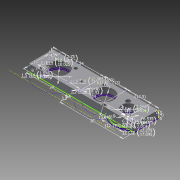
# Autodesk Inventor part: mount
Saved by Autodesk Inventor 2014 (Build 180170000, 170)
## iProperties
Created: 2013-09-13
Part Number: mount
Material: Generic
Document SubType Name: Modeling
Designer: Brandon
Density: 1 g/cm^3
Appearance: Default
Author: Brandon
Autodesk Inventor part; units mm, degrees
ref_plane "YZ Plane" through (0, 0, 0) normal (1, 0, 0) x (0, 1, 0)
ref_plane "XZ Plane" through (0, 0, 0) normal (0, 1, 0) x (-1, 0, 0)
ref_plane "XY Plane" through (0, 0, 0) normal (0, 0, 1) x (1, 0, 0)
sketch "Sketch1" plane through (0, 0, 0) normal (0, 0, 1) x (1, 0, 0)
  circle A0 centre (0, 0) radius 0.88
  circle A1 centre (-13, 0) radius 6.031
  line L0 (0, 7.8745) -> (0, -6.1255)
  line L1 (-24, -6.1255) -> (0, -6.1255)
  line L2 (-24, 7.8745) -> (-24, -6.1255)
  circle A2 centre (-13, 0) radius 5.1925
  line L3 (-13, 0) -> (-9.1435, 0) construction
  line L4 (-13, 0) -> (-13, 0) construction
  circle A3 centre (-8.099, 4.901) radius 0.8125
  circle A4 centre (-17.901, -4.901) radius 0.8125
  circle A5 centre (13, 0) radius 6.031
  circle A6 centre (13, 0) radius 5.1925
  line L5 (13, 0) -> (9.1435, 0) construction
  line L6 (13, 0) -> (13, 0) construction
  circle A7 centre (8.099, 4.901) radius 0.8125
  circle A8 centre (17.901, -4.901) radius 0.8125
  line L7 (13, 0) -> (-13, 0)
  circle A9 centre (26.5, 0) radius 4.5 construction
  circle A10 centre (26.5, 0) radius 8.6375
  line L8 (26.5, 0) -> (30.5894, 0) construction
  circle A11 centre (22.8938, 3.6062) radius 1.132
  circle A12 centre (30.1062, -3.6062) radius 1.132
  line L9 (0, -6.1255) -> (-0.0048, -7.7255) construction
  line L10 (-0.0048, -7.7255) -> (-19.5613, -7.6674) construction
  line L11 (-0.0048, -7.7255) -> (19.5518, -7.7836) construction
  circle A13 centre (13, 0) radius 9 construction
  circle A14 centre (26.5, 0) radius 2.5 construction
  circle A15 centre (26.5, 0) radius 3.2675
  line L12 (13, 0) -> (26.5, 0)
  line L13 (30.1062, -3.6062) -> (22.8938, 3.6062) construction
  line L14 (33.2882, -0.4243) -> (26.0757, 6.7882)
  line L15 (19.7118, 0.4243) -> (26.9243, -6.7882)
  arc A16 (26.9243, -6.7882) -> (33.2882, -0.4243) centre (30.1062, -3.6062) ccw
  arc A17 (26.0757, 6.7882) -> (19.7118, 0.4243) centre (22.8938, 3.6062) ccw
  circle A18 centre (26.5, 0) radius 7.7
  circle A19 centre (26.5, 0) radius 3.5
  line L16 (-24, 7.8745) -> (0, 7.8745)
  line L17 (36, 7.8745) -> (36, -6.1255)
  line L18 (20.4103, -6.1255) -> (32.5897, -6.1255) construction
  line L19 (-0.0048, -7.7255) -> (0.0011, -10.9255) construction
  line L20 (0.0011, -10.9255) -> (30.0189, -10.8709) construction
  line L21 (0.0011, -10.9255) -> (-29.9989, -10.9801) construction
  line L22 (0.0011, -10.9255) -> (30.001, -10.9255) construction
  circle A20 centre (0, 0) radius 4 construction
  line L23 (-13, 0) -> (-8.7354, 4.2646) construction
  line L24 (-13, 0) -> (-17.2646, -4.2646) construction
  line L25 (-8.7354, 4.2646) -> (-8.099, 4.901) construction
  line L26 (-17.2646, -4.2646) -> (-17.901, -4.901) construction
  line L27 (-17.2646, -4.2646) -> (-16.3646, -4.2646) construction
  circle A21 centre (13, 0) radius 12 construction
  circle A22 centre (-13, 0) radius 12 construction
  line L28 (1, 0) -> (-1, 0) construction
  line L29 (-19.031, 0) -> (-24, 0) construction
  line L30 (18.7135, -4.901) -> (18.7135, 10.099) construction
  line L31 (21.7618, 3.6062) -> (21.7618, -11.3938) construction
  line L32 (18.7135, -4.2879) -> (21.7618, -4.2879) construction
  line L33 (0, 7.8745) -> (36, 7.8745)
  line L34 (0, -6.1255) -> (36, -6.1255)
  dimension "d31" = 2
  dimension "d105" = 24
  dimension "d106" = 24
  dimension "d0" = 1.5
  dimension "d3" = 11.6
  dimension "d8" = 10
  dimension "d14" = 1.5
  dimension "d26" = 17
  dimension "d32" = 2
  dimension "d38" = 5
  dimension "d40" = 6.15
  dimension "d42" = 13
  dimension "d52" = 13.5
  dimension "d53" = 9
  dimension "d54" = 7
  dimension "d60" = 12.1794
  dimension "d81" = 1.6
  dimension "d86" = 3.2
  dimension "d87" = 45
  dimension "d88" = 10.2
  dimension "d89" = 8
  dimension "d91" = 0.9
  dimension "d92" = 135
  dimension "d98" = 14
  dimension "d103" = 18
  dimension "d104" = 9
  dimension "d107" = 2
  dimension "d108" = 4.969
  dimension "d114" = 3.0483
  dimension "d117" = 24
  dimension "d118" = 24
  dimension "d119" = 36
  constraints: 72 end point, 19 centre point, 15 coincident, 10 horizontal, 9 point on circle, 9 point on line, 7 collinear, 7 perpendicular, 6 symmetric about line, 6 tangent, 4 horizontal alignment, 3 equal length, 2 midpoint, 2 vertical, 1 equal radius, 1 parallel, 12 other
  measures "d38" diameter of A14
  measures "d42" distance of point (0, 0) A5.centre
  measures "d52" distance of L12.start L8.start
  measures "d53" diameter of A17
  measures "d54" diameter of A19
  measures "d60" distance of L18.start L18.end
  measures "d81" distance of L9.end L0.end
  measures "d86" distance of L9.end L19.end
  measures "d87" angle of L8 L13
  measures "d88" distance of L13.start L13.end
  measures "d89" diameter of A20
  measures "d91" distance of L24.end L26.end
  measures "d92" angle of L26 L27
  measures "d98" distance of L2.start L1.start
  measures "d103" diameter of A13
  measures "d104" diameter of A9
  measures "d107" distance of L28.start L28.end
  measures "d108" distance of L29.start L29.end
  measures "d114" distance of L32.start L32.end
  measures "d117" distance of L2.start L0.start
  measures "d118" distance of L1.start L0.end
  measures "d119" distance of L0.end L17.end
extrude "Extrusion5" add sketch "Sketch1" along normal blind 4 contours L7 L0 A0 | L7 A5 A10 L34 L0 A0 | A0 L0 L33 A17 A10 A5 L7 | A0 L0 L7 | L0 L7 A0 | A0 L0 L1 L2 L16 | A0 L7 L0 | L7 A6 A10 A5 | A5 A10 A6 L7 | A10 A17 A5 | A5 A18 L12 A6 A10 | A10 A6 L12 A18 A5 | A5 A18 L34 A10 | L33 A10 A17 | A17 A18 A5 | A17 A10 L33 A18 | A18 L12 A5 | A5 L12 L15 L34 A18 | A18 A17 L15 L12 A5 | A5 L12 A18 | A18 A17 L14 A16 L34 L15 | L33 L17 L34 A16 A10 | A10 A16 A18 A17 L33 | L34 A18 A16 A10 | A10 A16 L34 | A18 A16 L14 A17 | A1 picked at (19.4938, 5.5056) picked at (32.0861, -5.6911) picked at (33.2728, -5.8184)
extrude "Extrusion6" add sketch "Sketch1" along normal blind 0.6 contours A19
extrude "Extrusion7" add sketch "Sketch1" against normal blind 1 contours A18 L12 A5 | A5 L12 L15 L34 A18 | L34 L15 A16 A18 | A18 A17 L15 L12 A5 | A5 L12 A18 | A18 A17 L14 A16 L34 L15 | A16 L15 L34 A18 | A18 A16 L14 A17 | A19
extrude "Extrusion8" add sketch "Sketch1" against normal blind 2 contours L33 A10 A17 | A17 A10 L33 | A17 A10 L33 A18 | A17 L33 A10 | A16 A18 L34 A10 | A10 L34 A16 | A18 A17 L14 A16 L34 L15 | L34 A18 A16 A10 | A10 A16 L34 | A16 L15 L34 A18 | A19 picked at (19.4938, 5.5056) picked at (22.1766, 7.9288) picked at (23.7658, 7.9033) picked at (30.8384, -7.0828) picked at (32.0861, -5.6911) picked at (29.2006, -6.3392)
extrude "Extrusion9" cut sketch "Sketch1" against normal up to surface (1 mm away) from surface at -1 contours A10 A17 A5 | A5 A18 L12 A6 A10 | A10 A6 L12 A18 A5 | A5 A18 L34 A10 | A17 A18 A5 | A17 A10 L33 A18 | A6 L12 A10 | A18 L12 A5 | A5 L12 L15 L34 A18 | A10 L12 A6 | A17 L33 A10 | A10 L33 A17 | A18 A17 L15 L12 A5 | A5 L12 A18 | A18 A17 L14 A16 L34 L15 | A10 A16 A18 A17 L33 | L34 A18 A16 A10 | A18 A16 L14 A17 | A19 picked at (23.7658, 7.9033) picked at (27.6036, 8.0551) picked at (32.0861, -5.6911)
extrude "Extrusion10" cut sketch "Sketch1" against normal blind 2 contours L7 L0 A0 | L7 A5 A10 L34 L0 A0 | A0 L0 L33 A17 A10 A5 L7 | A0 L0 L7 | A10 A17 A5 | A5 A18 L34 A10 | L33 A10 A17 | A17 A18 A5 | A17 A10 L33 A18 | A5 L12 L15 L34 A18 | A18 A17 L15 L12 A5 | A18 A17 L14 A16 L34 L15 | L33 L17 L34 A16 A10 | A10 A16 A18 A17 L33 | L34 A18 A16 A10 | A10 A16 L34 | A18 A16 L14 A17 keep common part picked at (0.4122, 0.4122) picked at (0.4122, -0.4122) picked at (19.4938, 5.5056) picked at (32.0861, -5.6911) picked at (33.2728, -5.8184)
extrude "Extrusion11" add sketch "Sketch1" along normal blind 4 contours L7 L0 A0 | L7 A5 A10 L34 L0 A0 | A0 L0 L33 A17 A10 A5 L7 | A0 L0 L7 | L0 L7 A0 | A0 L0 L1 L2 L16 | A0 L7 L0 | L7 A6 A10 A5 | A5 A10 A6 L7 | A10 A17 A5 | A5 A18 L12 A6 A10 | A10 A6 L12 A18 A5 | A5 A18 L34 A10 | L33 A10 A17 | A17 A18 A5 | A17 A10 L33 A18 | A18 L12 A5 | A5 L12 L15 L34 A18 | A18 A17 L15 L12 A5 | A5 L12 A18 | A18 A17 L14 A16 L34 L15 | L33 L17 L34 A16 A10 | A10 A16 A18 A17 L33 | L34 A18 A16 A10 | A10 A16 L34 | A18 A16 L14 A17 | A1 picked at (19.4938, 5.5056) picked at (32.0861, -5.6911) picked at (33.2728, -5.8184)
extrude "Extrusion12" add sketch "Sketch1" against normal blind 1 contours A19
extrude "Extrusion13" add sketch "Sketch1" along normal blind 0.5 contours A19
extrude "Extrusion14" cut sketch "Sketch1" along normal blind 0.9 contours L7 A6 A10 A5 | A5 A10 A6 L7 | A5 A18 L12 A6 A10 | A10 A6 L12 A18 A5 | A18 L12 A5 | A5 L12 A18 | A1
extrude "Extrusion15" cut sketch "Sketch1" along normal blind 10 contours L7 L0 A0 | A0 L0 L7 | L0 L7 A0 | A0 L7 L0
sketch "Sketch2" plane through (21.4682, 7.8745, -2) normal (0, 1, 0) x (1, 0, 0)
  line L0 (-45.4682, -2) -> (-45.4682, -6) projected
  line L1 (14.5318, -2) -> (14.5318, -6) projected
  line L2 (1.4823, 0) -> (0, 0) projected
  line L3 (-45.4682, -4) -> (-43.4682, -4) construction
  line L4 (14.5318, -4) -> (12.5318, -4) construction
  circle A0 centre (-43.4682, -4) radius 1.25
  circle A1 centre (12.5318, -4) radius 1.25
  point P0 (-44.9213, -1)
  dimension "d120" = 60
  dimension "d121" = 4
  dimension "d122" = 4
  dimension "d123" = 2
  dimension "d124" = 2
  dimension "d126" = 2.5
  constraints: 4 end point, 2 centre point, 2 coincident, 2 midpoint, 1 collinear, 1 equal radius, 1 parallel
  measures "d120" distance of L1.end L0.end
  measures "d121" distance of L0.start L0.end
  measures "d122" distance of L1.start L1.end
  measures "d123" distance of L3.start L3.end
  measures "d124" distance of L4.start L4.end
  measures "d126" diameter of A0
extrude "Extrusion16" cut sketch "Sketch2" against normal blind 14 contours A0
extrude "Extrusion17" cut sketch "Sketch2" against normal blind 14 contours A1
body "Solid3"
